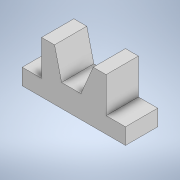
# Autodesk Inventor part: 零件1
Saved by Autodesk Inventor 2020 (Build 240168000, 168)
## iProperties
Created: 2023-11-09
Part Number: 零件1
Material: 常规
Document SubType Name: Modeling
Designer: Z
Density: 1 g/cm^3
Appearance: 默认
Author: Z
Autodesk Inventor part; units mm, degrees
ref_plane "YZ Plane" through (0, 0, 0) normal (1, 0, 0) x (0, 1, 0)
ref_plane "XZ Plane" through (0, 0, 0) normal (0, 1, 0) x (-1, 0, 0)
ref_plane "XY Plane" through (0, 0, 0) normal (0, 0, 1) x (1, 0, 0)
sketch "草图1" plane through (0, 0, 0) normal (0, 0, 1) x (1, 0, 0)
  line L0 (15.7018, 7.2486) -> (15.7018, 12.2486)
  line L1 (15.7018, 12.2486) -> (9.7018, 12.2486)
  line L2 (9.7018, 12.2486) -> (9.7018, 23.2486)
  line L3 (9.7018, 23.2486) -> (5.7018, 23.2486)
  line L4 (5.7018, 23.2486) -> (1.9029, 14.2486)
  line L5 (-16.2982, 7.2486) -> (-16.2982, 12.2486)
  line L6 (-16.2982, 12.2486) -> (-10.2982, 12.2486)
  line L7 (-10.2982, 12.2486) -> (-10.2982, 23.2486)
  line L8 (-10.2982, 23.2486) -> (-6.2982, 23.2486)
  line L9 (-6.2982, 23.2486) -> (-4.0971, 14.2486)
  line L10 (-16.2982, 7.2486) -> (15.7018, 7.2486)
  line L11 (1.9029, 14.2486) -> (-4.0971, 14.2486)
  dimension "d5" = 32
  dimension "d6" = 5
  dimension "d7" = 5
  dimension "d8" = 6
  dimension "d9" = 20
  dimension "d10" = 9
  dimension "d11" = 12
  dimension "d12" = 6
  dimension "d13" = 16
  dimension "d14" = 4
  dimension "d28" = 67.115
  constraints: 24 end point, 5 perpendicular, 2 horizontal, 1 collinear
  measures "d5" distance of L5.start L0.start
  measures "d6" distance of L0.start L0.end
  measures "d7" distance of L5.start L6.start
  measures "d8" distance of L4.end L9.end
  measures "d9" distance between parallel lines of L2 L7
  measures "d10" distance between parallel lines of L8 L11
  measures "d11" distance of L3.end L9.start
  measures "d12" distance between parallel lines of L0 L2
  measures "d13" distance between parallel lines of L10 L8
  measures "d14" distance of L9.start L8.start
  measures "d28" angle of L1 L4
sketch "草图2" plane through (0, 0, 0) normal (0, 0, 1) x (1, 0, 0)
  point P0 (0, 0)
extrude "拉伸1" add sketch "草图1" along normal blind 10
